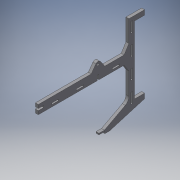
# Autodesk Inventor part: TrayPanelG
Saved by Autodesk Inventor 2017 (Build 210142000, 142)
## iProperties
Created: 2019-06-23
Part Number: TrayPanelG
Material: Generic
Document SubType Name: Modeling
Designer: DDeGo
Density: 1 g/cm^3
Appearance: Default
Author: DDeGo
Autodesk Inventor part; units mm, degrees
ref_plane "YZ Plane" through (0, 0, 0) normal (1, 0, 0) x (0, 1, 0)
ref_plane "XZ Plane" through (0, 0, 0) normal (0, 1, 0) x (-1, 0, 0)
ref_plane "XY Plane" through (0, 0, 0) normal (0, 0, 1) x (1, 0, 0)
sketch "Sketch1" plane through (0, 0, 0) normal (1, 0, 0) x (0, 1, 0)
  line L0 (0, 0) -> (8.6, 0)
  line L1 (8.6, 0) -> (8.6, -2.75)
  line L2 (8.6, -2.75) -> (15.6, -2.75)
  line L3 (15.6, -2.75) -> (66.85, 10.5)
  line L4 (66.85, 10.5) -> (66.85, 19.5)
  line L5 (66.85, 19.5) -> (51.85, 19.5)
  line L6 (51.85, 19.5) -> (51.85, 118.5)
  line L7 (51.85, 118.5) -> (66.85, 118.5)
  line L8 (66.85, 118.5) -> (66.85, 127.5)
  line L9 (43.85, 21) -> (8, 2)
  line L10 (8, 2) -> (0, 2)
  line L11 (0, 2) -> (0, 0)
  line L12 (0, 70) -> (0, 77)
  line L13 (0, 77) -> (-2.75, 77)
  line L14 (-2.75, 77) -> (-2.75, 70)
  line L15 (-2.75, 70) -> (-88.9, 70)
  line L16 (-88.9, 77.875) -> (-80.9, 77.875)
  line L17 (-80.9, 77.875) -> (-80.9, 75.125)
  line L18 (-80.9, 75.125) -> (-88.9, 75.125)
  line L19 (-88.9, 70) -> (-88.9, 75.125)
  line L20 (-88.9, 77.875) -> (-88.9, 83)
  line L21 (0, 70) -> (36.85, 70)
  line L22 (36.85, 70) -> (43.85, 59)
  line L23 (43.85, 94) -> (36.85, 83)
  line L24 (36.85, 83) -> (36.85, 70) construction
  line L25 (36.85, 83) -> (-88.9, 83)
  line L26 (43.85, 127.5) -> (43.85, 94)
  line L27 (43.85, 59) -> (43.85, 21)
  line L28 (43.85, 127.5) -> (66.85, 127.5)
  line L29 (-1.375, 77) -> (-1.375, 90) construction
  arc A0 (1.866, 92.3443) -> (-4.616, 92.3443) centre (-1.375, 90) ccw
  line L30 (-4.616, 92.3443) -> (-11.375, 83)
  line L31 (1.866, 92.3443) -> (8.625, 83)
  circle A1 centre (-1.375, 90) radius 1.5
  dimension "d0" = 2.75
  dimension "d1" = 8.6
  dimension "d2" = 7
  dimension "d3" = 2
  dimension "d4" = 43.25
  dimension "d6" = 15
  dimension "d7" = 99
  dimension "d8" = 9
  dimension "d14" = 19.5
  dimension "d16" = 8
  dimension "d25" = 9
  dimension "d27" = 2.75
  dimension "d29" = 8.6
  dimension "d31" = 97.5
  dimension "d32" = 2.75
  dimension "d33" = 8
  dimension "d34" = 7
  dimension "d35" = 13
  dimension "d36" = 8
  dimension "d37" = 8
  dimension "d38" = 7
  dimension "d39" = 35
  dimension "d42" = 83
  dimension "d56" = 8
  dimension "d57" = 3
  dimension "d58" = 7
  dimension "d59" = 10
  dimension "d61" = 38
  constraints: 64 end point, 14 perpendicular, 6 horizontal, 4 point on line, 3 equal length, 2 centre point, 2 coincident, 2 collinear, 2 point on circle, 2 tangent, 1 midpoint, 1 parallel, 1 vertical
  measures "d0" distance of L0.end L1.end
  measures "d1" distance of L0.start L0.end
  measures "d2" distance of L1.end L2.end
  measures "d3" distance of L10.end L0.start
  measures "d4" distance between parallel lines of L1 L6
  measures "d6" distance between parallel lines of L6 L4
  measures "d7" distance between parallel lines of L7 L5
  measures "d8" distance of L3.end L4.end
  measures "d14" distance from line of L0.end L5
  measures "d16" distance of L9.end L10.end
  measures "d25" distance of L7.end L8.end
  measures "d27" distance between parallel lines of L12 L14
  measures "d29" distance between parallel lines of L12 L1
  measures "d31" distance between parallel lines of L1 L20
  measures "d32" distance between parallel lines of L18 L16
  measures "d33" distance between parallel lines of L17 L19
  measures "d34" distance of L12.start L12.end
  measures "d35" distance between parallel lines of L25 L15
  measures "d36" distance between parallel lines of L6 L27
  measures "d37" distance between parallel lines of L6 L26
  measures "d38" distance between parallel lines of L24 L27
  measures "d39" distance of L23.start L22.end
  measures "d42" distance between parallel lines of L25 L0
  measures "d56" diameter of A0
  measures "d57" diameter of A1
  measures "d58" distance from line of L29.end L25
  measures "d59" distance from line of L29 L31.end
  measures "d61" distance of L22.end L9.start
extrude "Extrusion1" add sketch "Sketch1" along normal blind 4.3
sketch "Sketch2" plane through (4.3, 0, 0) normal (1, 0, 0) x (0, 0, -1)
  line L0 (-120.5, 48.225) -> (-105.5, 48.225)
  line L1 (-105.5, 48.225) -> (-105.5, 45.475)
  line L2 (-105.5, 45.475) -> (-120.5, 45.475)
  line L3 (-120.5, 45.475) -> (-120.5, 48.225)
  line L4 (-90.5, 48.225) -> (-75.5, 48.225)
  line L5 (-75.5, 48.225) -> (-75.5, 45.475)
  line L6 (-75.5, 45.475) -> (-90.5, 45.475)
  line L7 (-90.5, 45.475) -> (-90.5, 48.225)
  line L8 (-60.5, 48.225) -> (-45.5, 48.225)
  line L9 (-45.5, 48.225) -> (-45.5, 45.475)
  line L10 (-45.5, 45.475) -> (-60.5, 45.475)
  line L11 (-60.5, 45.475) -> (-60.5, 48.225)
  line L12 (-30.5, 48.225) -> (-15.5, 48.225)
  line L13 (-15.5, 48.225) -> (-15.5, 45.475)
  line L14 (-15.5, 45.475) -> (-30.5, 45.475)
  line L15 (-30.5, 45.475) -> (-30.5, 48.225)
  line L16 (-127.5, 66.85) -> (-127.5, 43.85) projected
  line L17 (-19.5, 51.85) -> (-118.5, 51.85) projected
  line L18 (-127.5, 43.85) -> (-94, 43.85) projected
  line L19 (-105.5, 46.85) -> (-104.169, 46.85) construction
  line L20 (-104.169, 46.85) -> (-104.169, 43.85) construction
  line L21 (-127.5, 43.85) -> (-94, 43.85) projected
  point P0 (0, 0)
  dimension "d43" = 7
  dimension "d44" = 2.75
  dimension "d46" = 15
  dimension "d47" = 30
  dimension "d48" = 30
  dimension "d49" = 15
  dimension "d50" = 15
  dimension "d51" = 15
  dimension "d52" = 30
  dimension "d72" = 3
  constraints: 36 end point, 8 parallel, 5 horizontal, 5 point on line, 4 perpendicular, 2 collinear, 1 midpoint, 1 vertical
  measures "d43" distance between parallel lines of L16 L3
  measures "d44" distance of L2.end L0.start
  measures "d46" distance between parallel lines of L3 L1
  measures "d47" distance between parallel lines of L7 L3
  measures "d48" distance between parallel lines of L7 L11
  measures "d49" distance of L5.end L6.end
  measures "d50" distance of L9.end L10.end
  measures "d51" distance of L13.end L14.end
  measures "d52" distance between parallel lines of L15 L11
  measures "d72" distance of L19.end L20.end
extrude "Extrusion2" cut sketch "Sketch2" against normal blind 10
fillet "Fillet1" radius 10 1 edges at (2.15, 43.85, 21)
sketch "Sketch3" plane through (4.3, 0, 0) normal (1, 0, 0) x (0, 0, -1)
  line L0 (-75, -22.75) -> (-73, -22.75)
  line L1 (-73, -22.75) -> (-73, -32.75)
  line L2 (-73, -32.75) -> (-75, -32.75)
  line L3 (-75, -32.75) -> (-75, -22.75)
  line L4 (-75, -58.9) -> (-73, -58.9)
  line L5 (-73, -58.9) -> (-73, -68.9)
  line L6 (-73, -68.9) -> (-75, -68.9)
  line L7 (-75, -68.9) -> (-75, -58.9)
  line L8 (-70, -88.9) -> (-70, -2.75) projected
  line L9 (-77.875, -80.9) -> (-75.125, -80.9) projected
  line L10 (-70, -2.75) -> (-77, -2.75) projected
  line L11 (-73, 20) -> (-75, 20)
  line L12 (-75, 20) -> (-75, 30)
  line L13 (-75, 30) -> (-73, 30)
  line L14 (-73, 30) -> (-73, 20)
  line L15 (-77, 0) -> (-70, 0) projected
  point P0 (0, 0)
  dimension "d62" = 10
  dimension "d63" = 2
  dimension "d64" = 3
  dimension "d65" = 12
  dimension "d66" = 20
  dimension "d69" = 20
  dimension "d70" = 10
  constraints: 24 end point, 6 parallel, 3 collinear, 3 horizontal, 3 perpendicular, 2 point on line
  measures "d62" distance of L6.end L4.start
  measures "d63" distance of L5.end L6.end
  measures "d64" distance between parallel lines of L8 L5
  measures "d65" distance between parallel lines of L9 L6
  measures "d66" distance between parallel lines of L10 L0
  measures "d69" distance between parallel lines of L15 L11
  measures "d70" distance of L13.end L11.start
extrude "Extrusion3" cut sketch "Sketch3" against normal blind 10
sketch "Sketch4" plane through (4.3, 0, 0) normal (1, 0, 0) x (0, 0, -1)
  line L0 (-19.5, 51.85) -> (-118.5, 51.85) projected
  line L1 (-77.875, 51.85) -> (-75.125, 51.85)
  line L2 (-75.125, 51.85) -> (-75.125, 49.85)
  line L3 (-75.125, 49.85) -> (-77.875, 49.85)
  line L4 (-77.875, 49.85) -> (-77.875, 51.85)
  line L5 (-77.875, -88.9) -> (-77.875, -80.9) projected
  line L6 (-75.125, -80.9) -> (-75.125, -88.9) projected
  line L7 (-90.5, 48.225) -> (-75.5, 48.225) projected
  point P0 (0, 0)
  dimension "d73" = 2
  dimension "d74" = 1.625
  constraints: 8 end point, 2 collinear, 2 parallel, 1 horizontal, 1 perpendicular, 1 point on line
  measures "d73" distance between parallel lines of L0 L3
  measures "d74" distance between parallel lines of L7 L3
extrude "Extrusion4" cut sketch "Sketch4" against normal blind 10
body "Solid1"
